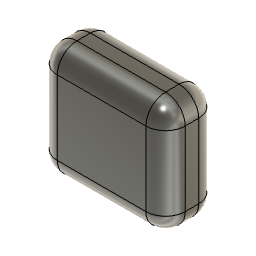
Airpod (Autodesk Fusion 360 design; units mm, degrees)
Autodesk Fusion 360 part; units mm, degrees
box "BoxPrimitive1" add length 46.2 width 52.1 height 21.5 placed x (0, 0, 1) y (1, 0, 0) z (0, 1, 0) at (0, 0, 0)
fillet "Fillet1" radius 8 6 faces at (52.1, 7.1667, 30.8) (17.3667, 7.1667, 46.2) (17.3667, 7.1667, 0) (0, 7.1667, 30.8) (34.7333, 0, 15.4) (34.7333, 21.5, 15.4)
